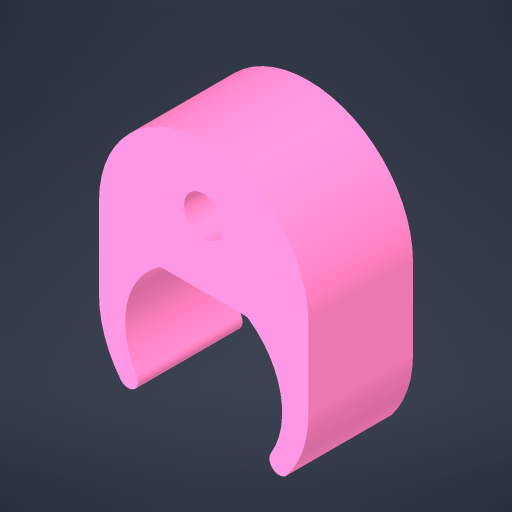
# Autodesk Inventor part: Y Stage Motor Clamp V5
Saved by Autodesk Inventor 2023.4 (Build 274418000, 418)
## iProperties
Created: 2024-05-29
Part Number: Y Stage Motor Clamp V5
Material: Generic
Document SubType Name: Modeling
Designer: xSibe
Density: 1 g/cm^3
Appearance: Plastic Pink
Author: xSibe
Autodesk Inventor part; units mm, degrees
ref_plane "YZ Plane" through (0, 0, 0) normal (1, 0, 0) x (0, 1, 0)
ref_plane "XZ Plane" through (0, 0, 0) normal (0, 1, 0) x (-1, 0, 0)
sketch "Sketch1" plane through (0, 0, 0) normal (0, 0, 1) x (1, 0, 0)
  line L0 (127.525, 5) -> (129.95, 5)
  line L1 (127.525, 15.075) -> (127.525, 5)
  line L2 (115.375, 15.075) -> (127.525, 15.075)
  line L3 (115.375, 5) -> (115.375, 15.075)
  line L4 (112.95, 5) -> (115.375, 5)
  line L5 (129.95, 5) -> (129.95, 25.025)
  line L6 (115.45, 10) -> (115.45, 6)
  arc A0 (115.45, 10) -> (118.000243, 5.090909) centre (121.45, 10) ccw
  arc A1 (118.000243, 5.090909) -> (118.287722, 5) centre (118.287722, 5.5) ccw
  line L7 (116.45, 5) -> (118.287722, 5)
  arc A2 (115.45, 6) -> (116.45, 5) centre (116.45, 6) ccw
  line L8 (118.287722, 15) -> (116.45, 15)
  arc A3 (118.287722, 15) -> (118.000243, 14.909091) centre (118.287722, 14.5) ccw
  arc A4 (118.000243, 14.909091) -> (115.45, 10) centre (121.45, 10) ccw
  line L9 (115.45, 14) -> (115.45, 10)
  arc A5 (116.45, 15) -> (115.45, 14) centre (116.45, 14) ccw
  line L10 (127.45, 10) -> (127.45, 14)
  arc A6 (127.45, 10) -> (124.899757, 14.909091) centre (121.45, 10) ccw
  arc A7 (124.899757, 14.909091) -> (124.612278, 15) centre (124.612278, 14.5) ccw
  line L11 (126.45, 15) -> (124.612278, 15)
  arc A8 (127.45, 14) -> (126.45, 15) centre (126.45, 14) ccw
  line L12 (124.612278, 5) -> (126.45, 5)
  arc A9 (124.612278, 5) -> (124.899757, 5.090909) centre (124.612278, 5.5) ccw
  arc A10 (124.899757, 5.090909) -> (127.45, 10) centre (121.45, 10) ccw
  line L13 (127.45, 6) -> (127.45, 10)
  arc A11 (126.45, 5) -> (127.45, 6) centre (126.45, 6) ccw
  arc A12 (118.000243, 5.090909) -> (118.287722, 5) centre (118.287722, 5.5) ccw
  arc A13 (118.000243, 14.909091) -> (118.000243, 5.090909) centre (121.45, 10) ccw
  arc A14 (118.287722, 15) -> (118.000243, 14.909091) centre (118.287722, 14.5) ccw
  line L14 (118.287722, 15) -> (124.612278, 15)
  arc A15 (124.899757, 14.909091) -> (124.612278, 15) centre (124.612278, 14.5) ccw
  arc A16 (124.899757, 5.090909) -> (124.899757, 14.909091) centre (121.45, 10) ccw
  arc A17 (124.612278, 5) -> (124.899757, 5.090909) centre (124.612278, 5.5) ccw
  line L15 (124.612278, 5) -> (118.287722, 5)
  line L16 (127.45, 15.075) -> (129.45, 15.075)
  line L17 (129.45, 15.075) -> (129.45, 5)
  line L18 (129.45, 5) -> (127.45, 5)
  line L19 (127.45, 5) -> (127.45, 15.075)
  line L20 (121.45, 10) -> (121.45, 5)
  arc A18 (127.157107, 5.292893) -> (129.45, 10.828427) centre (121.621573, 10.828427) ccw
  line L21 (115.45, 15.075) -> (113.45, 15.075)
  line L22 (113.45, 15.075) -> (113.45, 5)
  line L23 (113.45, 5) -> (115.45, 5)
  line L24 (115.45, 5) -> (115.45, 15.075)
  arc A19 (113.45, 10.828427) -> (115.742893, 5.292893) centre (121.278427, 10.828427) ccw
  line L25 (121.45, 25) -> (121.45, 15)
  circle A20 centre (121.45, 20) radius 1.5
  circle A21 centre (121.45, 20) radius 3
  line L26 (129.45, 15) -> (113.45, 15)
  line L27 (113.45, 15) -> (113.45, 25)
  line L28 (113.45, 25) -> (129.45, 25)
  line L29 (129.45, 25) -> (129.45, 15)
  arc A22 (129.45, 17) -> (121.45, 25) centre (121.45, 17) ccw
  arc A23 (121.45, 25) -> (113.45, 17) centre (121.45, 17) ccw
  circle A24 centre (121.45, 20) radius 1.4375
  line L30 (129.95, 25.025) -> (112.95, 25.025)
  line L31 (112.95, 25.025) -> (112.95, 5)
  point P0 (0, 0)
  point P1 (112.95, 16.464466)
  point P2 (115.742893, 5.292893)
  point P3 (127.45, 5.602175)
  point P4 (115.45, 5.602175)
  point P5 (115.45, 15)
  point P6 (127.45, 15)
  dimension "d0" = 2
  dimension "d2" = 3
  dimension "d3" = 6
  dimension "d10" = 10
  constraints: 28 end point, 9 point on circle, 8 point on line, 7 symmetric about line, 6 centre point, 6 tangent, 4 midpoint, 4 parallel, 3 collinear, 2 perpendicular, 1 coincident, 1 horizontal, 1 vertical, 1 other
  measures "d0" distance of L17.end L18.end
  measures "d2" diameter of A20
  measures "d3" diameter of A21
  measures "d10" distance of L26.end L27.end
ref_plane "Work Plane1" through (127.525, 15.075, -31.525) normal (0, 0, -1) x (-1, 0, 0)
sketch "Sketch1 outline for Extrusion1" plane through (0, 0, 0) normal (0, 0, 1) x (1, 0, 0)
  arc A0 (124.612278, 15) -> (124.899757, 14.909091) centre (124.612278, 14.5) cw
  line L0 (118.287722, 15) -> (124.612278, 15)
  arc A1 (124.899757, 14.909091) -> (127.45, 10) centre (121.45, 10) cw
  arc A2 (118.000243, 14.909091) -> (118.287722, 15) centre (118.287722, 14.5) cw
  arc A3 (127.45, 10) -> (124.899757, 5.090909) centre (121.45, 10) cw
  arc A4 (115.45, 10) -> (118.000243, 14.909091) centre (121.45, 10) cw
  arc A5 (124.899757, 5.090909) -> (124.612278, 5) centre (124.612278, 5.5) cw
  arc A6 (118.000243, 5.090909) -> (115.45, 10) centre (121.45, 10) cw
  line L1 (124.612278, 5) -> (126.45, 5)
  arc A7 (118.287722, 5) -> (118.000243, 5.090909) centre (118.287722, 5.5) cw
  arc A8 (126.45, 5) -> (127.157107, 5.292893) centre (126.45, 6) ccw
  line L2 (116.45, 5) -> (118.287722, 5)
  arc A9 (127.157107, 5.292893) -> (129.45, 10.828427) centre (121.621573, 10.828427) ccw
  arc A10 (115.742893, 5.292893) -> (116.45, 5) centre (116.45, 6) ccw
  line L3 (129.45, 10.828427) -> (129.45, 15.075)
  arc A11 (113.45, 10.828427) -> (115.742893, 5.292893) centre (121.278427, 10.828427) ccw
  line L4 (129.45, 15.075) -> (129.45, 17)
  line L5 (113.45, 15.075) -> (113.45, 10.828427)
  arc A12 (129.45, 17) -> (121.45, 25) centre (121.45, 17) ccw
  line L6 (113.45, 17) -> (113.45, 15.075)
  arc A13 (121.45, 25) -> (113.45, 17) centre (121.45, 17) ccw
  circle A14 centre (121.45, 20) radius 1.5
extrude "Extrusion1" add sketch "Sketch1 outline for Extrusion1" against normal blind 6 from surface at -31.525
fillet "Fillet1" radius 0.75 4 edges at (124.8998, 5.0909, -34.525) (118.0002, 5.0909, -34.525) (124.6123, 5, -34.525) (118.2877, 5, -34.525)
sketch "Sketch2" plane through (121.45, 14.820968, -37.525) normal (0, 0, -1) x (-1, 0, 0)
  arc A0 (6.362384, -8.784005) -> (8, -3.992541) centre (0.171573, -3.992541) ccw
  line L0 (8, 2.179032) -> (8, -3.992541)
  line L1 (-8, -3.992541) -> (-8, 2.179032)
  arc A1 (-8, -3.992541) -> (-6.362384, -8.784005) centre (-0.171573, -3.992541) ccw
  arc A2 (-3.449757, 0.088123) -> (-5.128245, -7.935627) centre (0, -4.820968) ccw
  arc A3 (-3.162278, 0.179032) -> (-3.449757, 0.088123) centre (-3.162278, -0.320968) ccw
  arc A4 (3.449757, 0.088123) -> (3.162278, 0.179032) centre (3.162278, -0.320968) ccw
  arc A5 (5.128245, -7.935627) -> (3.449757, 0.088123) centre (0, -4.820968) ccw
  circle A6 centre (0, 5.179032) radius 3
  line L2 (3.162278, 0.179032) -> (-3.162278, 0.179032)
  circle A7 centre (0, 5.179032) radius 1.5
  arc A8 (8, 2.179032) -> (-8, 2.179032) centre (0, 2.179032) ccw
  arc A9 (5.128245, -7.935627) -> (6.362384, -8.784005) centre (5.769275, -8.32496) ccw
  arc A10 (-6.362384, -8.784005) -> (-5.128245, -7.935627) centre (-5.769275, -8.32496) ccw
  point P0 (121.45, -14.820968)
  dimension "d7" = 6
  constraints: 1 centre point, 1 coincident
  measures "d7" diameter of A6
sketch "Sketch2 outline for Extrusion2" plane through (121.45, 14.820968, -37.525) normal (0, 0, -1) x (-1, 0, 0)
  arc A0 (5.128245, -7.935627) -> (6.362384, -8.784005) centre (5.769275, -8.32496) ccw
  arc A1 (3.449757, 0.088123) -> (5.128245, -7.935627) centre (0, -4.820968) cw
  arc A2 (6.362384, -8.784005) -> (8, -3.992541) centre (0.171573, -3.992541) ccw
  arc A3 (3.162278, 0.179032) -> (3.449757, 0.088123) centre (3.162278, -0.320968) cw
  line L0 (8, -3.992541) -> (8, 2.179032)
  line L1 (-3.162278, 0.179032) -> (3.162278, 0.179032)
  arc A4 (8, 2.179032) -> (-8, 2.179032) centre (0, 2.179032) ccw
  arc A5 (-3.449757, 0.088123) -> (-3.162278, 0.179032) centre (-3.162278, -0.320968) cw
  line L2 (-8, 2.179032) -> (-8, -3.992541)
  arc A6 (-5.128245, -7.935627) -> (-3.449757, 0.088123) centre (0, -4.820968) cw
  arc A7 (-8, -3.992541) -> (-6.362384, -8.784005) centre (-0.171573, -3.992541) ccw
  arc A8 (-6.362384, -8.784005) -> (-5.128245, -7.935627) centre (-5.769275, -8.32496) ccw
  circle A9 centre (0, 5.179032) radius 3
extrude "Extrusion2" add sketch "Sketch2 outline for Extrusion2" along normal blind 2
body "Solid1"
